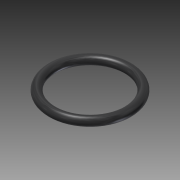
# Autodesk Inventor part: OringSmall
Saved by Autodesk Inventor 2014 SP2 (Build 180246200, 246)
## iProperties
Created: 2015-09-18
Part Number: OringSmall
Material: Rubber
Document SubType Name: Modeling
Designer: Lukasz Szmit
Density: 0.93 g/cm^3
Appearance: Rubber - Black - Version 1.1
Mass: 0.139996 g
Surface Area: 3.16913 cm^2
Volume: 0.150534 cm^3
Author: Lukasz Szmit
Autodesk Inventor part; units mm, degrees
ref_plane "YZ Plane" through (0, 0, 0) normal (1, 0, 0) x (0, 1, 0)
ref_plane "XZ Plane" through (0, 0, 0) normal (0, 1, 0) x (-1, 0, 0)
ref_plane "XY Plane" through (0, 0, 0) normal (0, 0, 1) x (1, 0, 0)
sketch "Sketch2" plane through (0, 0, 0) normal (0, 1, 0) x (-1, 0, 0)
  circle A0 centre (8.45, 4.95) radius 0.95
  line L0 (0, -1.18) -> (0, 7.08) projected
  point P0 (0, 0)
  dimension "d4" = 8.45
  dimension "d4" = 8.45
  constraints: 1 centre point
  measures "d4" horizontal distance of point (0, 0) A0.centre
revolve "Revolution2" add sketch "Sketch2" angle 360 about axis through (0, 0, -10) along (0, 0, 1)
body "Solid2"
